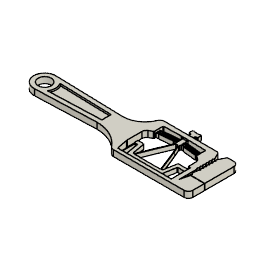
Final_BinaryStiffnessWrench (Autodesk Fusion 360 design; units mm, degrees)
Autodesk Fusion 360 part; units mm, degrees
note: some values were not read from the file. Set by a fixed rule: which sketch regions a step uses.
(part 1 of 3)
sketch "Sketch1" plane through (0, 0, 0) normal (0, 0, 1) x (1, 0, 0)
  arc A0 (89.3732, 10.2649) -> (113.1229, 26.2409) centre (89.45, 35.7917) ccw
  arc A1 (11.704, 12.452) -> (11.9433, -12.5645) centre (11.002, -0.0641) ccw
  arc A2 (112.7407, -25.7315) -> (80.6073, -9.9709) centre (80.1774, -51.4853) ccw
  line L0 (176.5, -1.6298) -> (183.1113, -1.6298)
  line L1 (184, 5.6067) -> (184, 5.6087)
  line L2 (149.0449, 22.5392) -> (149.0454, 22.5392)
  line L3 (184.0001, 9.0708) -> (184.0001, 9.073)
  line L4 (172.4, -5.8471) -> (172.4, -5.8496)
  line L5 (177.088, -7.1298) -> (177.088, -23.1298)
  line L6 (177.588, -23.1298) -> (177.588, -7.1298)
  line L7 (202.169, -22.6429) -> (202.2039, -9.25)
  circle A3 centre (11.002, -0.0641) radius 7.5
  line L8 (11.9433, -12.5645) -> (80.6073, -9.9709)
  line L9 (202.156, -8.9998) -> (202.156, 24.3702)
  line L10 (89.3732, 10.2649) -> (11.704, 12.452)
  line L11 (121.2059, -23.1298) -> (121.2059, -7.1298)
  line L12 (171.2956, -5.8495) -> (171.2956, -5.8471)
  line L13 (184, 2.1426) -> (184, 2.1446)
  line L14 (186.578, -8.932) -> (202.156, -8.9998)
  line L15 (184.001, 12.5353) -> (184.001, 12.5385)
  line L16 (186.1089, -9.5607) -> (182.6828, -23.2512)
  line L17 (202.2039, -9.25) -> (186.5961, -9.1821)
  line L18 (177.588, -28.2111) -> (177.588, -28.4)
  spline S0 degree 3 poles (139.0353, -28.3354) (139.0353, -28.3354) (139.0354, -28.3354) (139.0354, -28.3354) knots 113.159202 113.159202 113.159202 113.159202 113.159512 113.159512 113.159512 113.159512
  line L19 (169.6572, 23.9078) -> (150.1207, 24.3589)
  line L20 (149.6323, 24.8588) -> (149.6323, 29.3702)
  line L21 (149.6323, 29.3702) -> (178.1615, 29.3702)
  line L22 (178.088, -23.6298) -> (182.1978, -23.6298)
  line L23 (169.2352, -6.6298) -> (176.588, -6.6298)
  line L24 (121.7059, -6.6298) -> (122.93, -6.6298)
  line L25 (120.2059, -2.6298) -> (126.2864, -2.6298)
  line L26 (126.0097, -21.7167) -> (123.4224, -7.043)
  line L27 (168.7428, -7.043) -> (166.1554, -21.7167)
  spline S1 degree 5 poles (159.9652, -15.6911) (159.8529, -15.3927) (159.4459, -14.3123) (158.7459, -12.4635) (157.7568, -9.8732) (156.4844, -6.5848) (155.0461, -2.9325) (153.6231, 0.6091) (152.4351, 3.5002) (151.5369, 5.6459) (150.9212, 7.0983) (150.5836, 7.8891) (150.5222, 8.0328) knots 0.061951 0.061951 0.061951 0.061951 0.061951 0.061951 0.1 0.2 0.3 0.4 0.5 0.6 0.7 0.722257 0.722257 0.722257 0.722257 0.722257 0.722257
  line L28 (132.1188, -18.1298) -> (160.1605, -18.1298)
  line L29 (159.9652, -15.6911) -> (160.6285, -17.4538)
  line L30 (126.5021, -22.1298) -> (165.663, -22.1298)
  line L31 (119.7059, -3.1298) -> (119.7059, -6.1298)
  line L32 (120.2059, -23.6298) -> (118.121, -23.6298)
  line L33 (121.7059, -23.6298) -> (176.588, -23.6298)
  line L34 (120.7059, -7.1298) -> (120.7059, -23.1298)
  line L35 (170.1456, 15.3966) -> (193.3883, 15.3966) construction
  line L36 (146.1323, 17.0362) -> (146.1323, 33.8702) construction
  line L37 (170.1456, 15.8966) -> (192.9161, 15.8966) construction
  line L38 (170.1456, 17.3966) -> (193.3497, 17.3966) construction
  line L39 (170.1456, 17.2165) -> (170.1456, 16.1187)
  line L40 (170.1456, 17.8966) -> (193.2684, 17.8966) construction
  line L41 (170.1456, 18.1187) -> (170.1456, 19.2165)
  line L42 (186.7149, 19.4345) -> (191.4009, 19.4345) construction
  line L43 (170.1456, 20.1187) -> (170.1456, 23.408)
  line L44 (148.6323, 17.4356) -> (148.6323, 15.55)
  line L45 (148.6323, 19.4356) -> (148.6323, 18.3378)
  line L46 (148.6323, 33.3702) -> (148.6323, 22.3378)
  line L47 (148.6323, 21.4356) -> (148.6323, 20.3378)
  line L48 (170.1456, 15.2165) -> (170.1456, 13.9739)
  line L49 (170.6456, 13.1079) -> (173.5, 11.4599)
  spline S2 degree 5 poles (130.7595, -17.6378) (131.012, -16.9513) (131.5314, -15.5453) (132.3224, -13.424) (133.3923, -10.5941) (134.7528, -7.0662) (136.1486, -3.5243) (137.5684, -0.0041) (139.0131, 3.4934) (140.482, 6.9691) (141.8006, 10.0246) (142.8329, 12.3782) (143.5692, 14.0387) (144.0034, 15.0117) (144.1323, 15.3) knots 0.004792 0.004792 0.004792 0.004792 0.004792 0.004792 0.1 0.2 0.3 0.4 0.5 0.6 0.7 0.8 0.9 0.94214 0.94214 0.94214 0.94214 0.94214 0.94214
  spline S3 degree 5 poles (144.9323, 15.3) (144.7729, 14.9268) (144.3238, 13.8732) (143.5856, 12.1354) (142.5604, 9.7063) (141.2507, 6.5745) (139.8173, 3.108) (138.3903, -0.385) (136.9701, -3.9054) (135.5564, -7.4521) (134.2095, -10.8681) (133.1481, -13.5859) (132.3693, -15.5934) (131.871, -16.8829) (131.6523, -17.4499) knots 0.045074 0.045074 0.045074 0.045074 0.045074 0.045074 0.1 0.2 0.3 0.4 0.5 0.6 0.7 0.8 0.9 0.978339 0.978339 0.978339 0.978339 0.978339 0.978339
  spline S4 degree 3 poles (150.5222, 8.0328) (150.3157, 8.4943) (150.1094, 8.9559) (149.9035, 9.4176) (149.4682, 10.3932) (149.0343, 11.3694) (148.603, 12.3469) (148.2003, 13.2596) (147.7999, 14.1733) (147.4174, 15.0945) (147.3889, 15.163) (147.3606, 15.2315) (147.3323, 15.3) knots -96.269727 -96.269727 -96.269727 -96.269727 -93.23622 -93.23622 -93.23622 -86.826165 -86.826165 -86.826165 -80.841267 -80.841267 -80.841267 -80.396364 -80.396364 -80.396364 -80.396364
  line L50 (143.6323, 33.3702) -> (143.6323, 22.3378)
  line L51 (143.6323, 21.4356) -> (143.6323, 20.3378)
  line L52 (143.6323, 19.4356) -> (143.6323, 18.3378)
  line L53 (143.6323, 17.4356) -> (143.6323, 15.55)
  line L54 (122.1189, 17.2165) -> (122.1189, 16.1187)
  line L55 (122.1189, 18.1187) -> (122.1189, 19.2165)
  line L56 (122.1189, 20.1187) -> (122.1189, 23.408)
  line L57 (122.1189, 15.2165) -> (122.1189, 13.9739)
  line L58 (142.6323, 29.3702) -> (117.7597, 29.3702)
  line L59 (143.8823, 15.3) -> (144.1323, 15.3)
  line L60 (144.9323, 15.3) -> (147.3323, 15.3)
  line L61 (148.1323, 15.3) -> (148.3823, 15.3)
  line L62 (130.7595, -17.6378) -> (129.7718, -17.6378)
  line L63 (129.2794, -17.2246) -> (126.7788, -3.043)
  line L64 (162.9139, -17.0652) -> (165.3864, -3.043)
  line L65 (165.8788, -2.6298) -> (184.9592, -2.6298)
  line L66 (185.4592, 0) -> (185.4592, -2.1298)
  line L67 (117.6907, 10.8399) -> (121.6189, 13.1079)
  line L68 (151.6323, 22.1424) -> (167.1456, 20.5119)
  line L69 (151.6323, 21.0424) -> (167.1456, 19.4119)
  line L70 (151.6323, 20.1424) -> (167.1456, 18.5119)
  line L71 (151.6323, 19.0424) -> (167.1456, 17.4119)
  line L72 (151.6323, 18.1424) -> (167.1456, 16.5119)
  line L73 (151.6323, 17.0424) -> (167.1456, 15.4119)
  line L74 (169.9247, 19.9198) -> (167.3247, 20.1931)
  line L75 (151.4114, 21.8656) -> (148.8114, 22.1389)
  line L76 (169.9665, 19.4154) -> (167.3665, 19.6887)
  line L77 (151.4532, 21.3612) -> (148.8532, 21.6345)
  line L78 (151.6323, 22.1424) -> (151.6323, 22.0645)
  line L79 (151.6323, 21.1623) -> (151.6323, 21.0424)
  line L80 (151.6323, 20.1424) -> (151.6323, 20.0645)
  line L81 (151.6323, 19.1623) -> (151.6323, 19.0424)
  line L82 (169.9665, 17.4154) -> (167.3665, 17.6887)
  line L83 (151.4532, 19.3612) -> (148.8532, 19.6345)
  line L84 (169.9247, 17.9198) -> (167.3247, 18.1931)
  line L85 (151.4114, 19.8656) -> (148.8114, 20.1389)
  line L86 (151.6323, 18.1424) -> (151.6323, 18.0645)
  line L87 (151.6323, 17.1623) -> (151.6323, 17.0424)
  line L88 (169.9665, 15.4154) -> (167.3665, 15.6887)
  line L89 (151.4532, 17.3612) -> (148.8532, 17.6345)
  line L90 (169.9247, 15.9198) -> (167.3247, 16.1931)
  line L91 (151.4114, 17.8656) -> (148.8114, 18.1389)
  line L92 (167.1456, 20.5119) -> (167.1456, 20.392)
  line L93 (167.1456, 19.4898) -> (167.1456, 19.4119)
  line L94 (167.1456, 18.5119) -> (167.1456, 18.392)
  line L95 (167.1456, 17.4898) -> (167.1456, 17.4119)
  line L96 (167.1456, 16.5119) -> (167.1456, 16.392)
  line L97 (167.1456, 15.4898) -> (167.1456, 15.4119)
  line L98 (140.6323, 17.1623) -> (140.6323, 17.2225)
  line L99 (140.6323, 21.2524) -> (140.6323, 21.2225)
  line L100 (140.7218, 19.3518) -> (143.4114, 19.6345)
  line L101 (140.6323, 19.8424) -> (143.4532, 20.1389)
  line L102 (140.6323, 17.9203) -> (140.6323, 17.8424)
  line L103 (140.4532, 17.0236) -> (125.3398, 15.4351)
  line L104 (122.3398, 15.9198) -> (125.1189, 16.2119)
  line L105 (140.6323, 19.2524) -> (140.6323, 19.2225)
  line L106 (140.4532, 19.0236) -> (125.3398, 17.4351)
  line L107 (140.4532, 21.0236) -> (125.3398, 19.4351)
  line L108 (140.6323, 21.8424) -> (143.4532, 22.1389)
  line L109 (125.1189, 17.7119) -> (125.1189, 17.634)
  line L110 (122.3398, 19.9198) -> (125.0294, 20.2025)
  line L111 (140.7218, 21.3518) -> (143.4114, 21.6345)
  line L112 (140.8114, 17.3612) -> (143.4114, 17.6345)
  line L113 (125.1189, 15.7119) -> (125.1189, 15.634)
  line L114 (122.298, 17.4154) -> (125.1189, 17.7119)
  line L115 (140.4114, 22.1192) -> (125.298, 20.5307)
  line L116 (140.4114, 20.1192) -> (125.298, 18.5307)
  line L117 (140.4114, 18.1192) -> (125.298, 16.5307)
  line L118 (122.3398, 17.9198) -> (125.1189, 18.2119)
  line L119 (125.1189, 16.3318) -> (125.1189, 16.2119)
  line L120 (140.6323, 17.8424) -> (143.4532, 18.1389)
  line L121 (122.298, 19.4154) -> (125.1189, 19.7119)
  line L122 (125.1189, 18.3318) -> (125.1189, 18.2119)
  line L123 (125.1189, 19.7119) -> (125.1189, 19.634)
  line L124 (140.6323, 19.9203) -> (140.6323, 19.8424)
  line L125 (122.298, 15.4154) -> (125.1189, 15.7119)
  line L126 (125.1189, 20.3318) -> (125.1189, 20.3019)
  line L127 (140.6323, 21.9203) -> (140.6323, 21.8424)
  line L128 (115.1907, 6.5098) -> (115.1907, -10.1247)
  line L129 (117.6301, -23.2247) -> (115.2816, -11.0735)
  line L130 (178.088, -6.6298) -> (185.5859, -6.6298)
  line L131 (186.0859, -7.132) -> (186.0802, -8.4298)
  line L132 (116.6624, -27.6298) -> (197.169, -27.6298)
  line L133 (142.6323, 29.3702) -> (142.6323, 24.8588)
  line L134 (142.1438, 24.3589) -> (122.6074, 23.9078)
  line L135 (162.4215, -17.4784) -> (161.7176, -17.4784)
  spline S5 degree 5 poles (148.1323, 15.3) (148.4158, 14.6516) (148.9812, 13.354) (149.8244, 11.4057) (150.9388, 8.8038) (152.3141, 5.5444) (153.6703, 2.2771) (155.0058, -0.9987) (156.3196, -4.2834) (157.6127, -7.5765) (158.8598, -10.8079) (159.8388, -13.3845) (160.5594, -15.3025) (161.0282, -16.559) (161.2489, -17.1526) knots 0 0 0 0 0 0 0.1 0.2 0.3 0.4 0.5 0.6 0.7 0.8 0.9 0.989467 0.989467 0.989467 0.989467 0.989467 0.989467
  line L136 (190.889, 29.3702) -> (197.156, 29.3702)
  line L137 (183.6113, 17.3326) -> (182.6113, 15.6006)
  line L138 (182.6113, 15.6006) -> (183.6113, 13.8685)
  line L139 (183.6113, 13.8685) -> (182.6113, 12.1365)
  line L140 (182.6113, 12.1365) -> (183.6113, 10.4044)
  line L141 (183.6113, 10.4044) -> (182.6113, 8.6724)
  line L142 (182.6113, 8.6724) -> (183.6113, 6.9403)
  line L143 (183.6113, 6.9403) -> (182.6113, 5.2083)
  line L144 (182.6113, 5.2083) -> (183.6113, 3.4762)
  line L145 (183.6113, 3.4762) -> (182.6113, 1.7442)
  line L146 (182.6113, 1.7442) -> (183.6113, 0.0121)
  line L147 (183.6113, 0.0121) -> (183.6113, -1.1298)
  line L148 (183.6113, 17.3326) -> (182.6113, 19.0647)
  line L149 (183.6113, 17.3326) -> (185.8426, 17.3326) construction
  line L150 (182.6113, 19.0647) -> (183.6113, 20.7967)
  line L151 (182.6113, 19.0647) -> (184.8426, 19.0647) construction
  line L152 (183.6113, 20.7967) -> (179.9574, 28.2505)
  line L153 (176, 7.1298) -> (176, -1.1298)
  line L154 (184.5253, -0.9908) -> (184.5253, 23.394) construction
  line L155 (186.4393, 19.0647) -> (185.4393, 20.7967)
  line L156 (185.4393, 20.7967) -> (189.0932, 28.2505)
  line L157 (185.4393, 17.3326) -> (186.4393, 19.0647)
  line L158 (185.4393, 17.3326) -> (186.4393, 15.6006)
  line L159 (186.4393, 15.6006) -> (185.4393, 13.8685)
  line L160 (185.4393, 13.8685) -> (186.4393, 12.1365)
  line L161 (186.4393, 12.1365) -> (185.4393, 10.4044)
  line L162 (185.4393, 10.4044) -> (186.4393, 8.6724)
  line L163 (186.4393, 8.6724) -> (185.4393, 6.9403)
  line L164 (185.4393, 6.9403) -> (186.4393, 5.2083)
  line L165 (186.4393, 5.2083) -> (185.4393, 3.4762)
  line L166 (185.4393, 3.4762) -> (186.4393, 1.7442)
  line L167 (186.4393, 1.7442) -> (185.4592, 0.0467)
  line L168 (185.4592, 0) -> (185.4592, 0.0467)
  arc A4 (122.6074, 23.9078) -> (122.1189, 23.408) centre (122.6189, 23.408) ccw
  arc A5 (170.1456, 23.408) -> (169.6572, 23.9078) centre (169.6456, 23.408) ccw
  arc A6 (170.1456, 13.9739) -> (170.6456, 13.1079) centre (171.1456, 13.9739) ccw
  arc A7 (176, 7.1298) -> (173.5, 11.4599) centre (171, 7.1298) ccw
  arc A8 (121.6189, 13.1079) -> (122.1189, 13.9739) centre (121.1189, 13.9739) ccw
  arc A9 (117.6907, 10.8399) -> (115.1907, 6.5098) centre (120.1907, 6.5098) ccw
  arc A10 (117.6301, -23.2247) -> (118.121, -23.6298) centre (118.121, -23.1298) ccw
  arc A11 (120.2059, -23.6298) -> (120.7059, -23.1298) centre (120.2059, -23.1298) ccw
  arc A12 (121.2059, -23.1298) -> (121.7059, -23.6298) centre (121.7059, -23.1298) ccw
  arc A13 (176.588, -23.6298) -> (177.088, -23.1298) centre (176.588, -23.1298) ccw
  arc A14 (177.588, -23.1298) -> (178.088, -23.6298) centre (178.088, -23.1298) ccw
  arc A15 (182.1978, -23.6298) -> (182.6828, -23.2512) centre (182.1978, -23.1298) ccw
  arc A16 (178.088, -6.6298) -> (177.588, -7.1298) centre (178.088, -7.1298) ccw
  arc A17 (177.088, -7.1298) -> (176.588, -6.6298) centre (176.588, -7.1298) ccw
  arc A18 (169.2352, -6.6298) -> (168.7428, -7.043) centre (169.2352, -7.1298) ccw
  arc A19 (165.663, -22.1298) -> (166.1554, -21.7167) centre (165.663, -21.6298) ccw
  arc A20 (165.8788, -2.6298) -> (165.3864, -3.043) centre (165.8788, -3.1298) ccw
  arc A21 (162.4215, -17.4784) -> (162.9139, -17.0652) centre (162.4215, -16.9784) ccw
  arc A22 (161.2489, -17.1526) -> (161.7176, -17.4784) centre (161.7176, -16.9784) ccw
  arc A23 (160.1605, -18.1298) -> (160.6285, -17.4538) centre (160.1605, -17.6298) ccw
  arc A24 (131.6523, -17.4499) -> (132.1188, -18.1298) centre (132.1188, -17.6298) ccw
  arc A25 (129.2794, -17.2246) -> (129.7718, -17.6378) centre (129.7718, -17.1378) ccw
  arc A26 (126.7788, -3.043) -> (126.2864, -2.6298) centre (126.2864, -3.1298) ccw
  arc A27 (120.2059, -2.6298) -> (119.7059, -3.1298) centre (120.2059, -3.1298) ccw
  arc A28 (119.7059, -6.1298) -> (120.2059, -6.6298) centre (120.2059, -6.1298) ccw
  arc A29 (120.7059, -7.1298) -> (120.2059, -6.6298) centre (120.2059, -7.1298) ccw
  arc A30 (121.7059, -6.6298) -> (121.2059, -7.1298) centre (121.7059, -7.1298) ccw
  arc A31 (123.4224, -7.043) -> (122.93, -6.6298) centre (122.93, -7.1298) ccw
  arc A32 (126.0097, -21.7167) -> (126.5021, -22.1298) centre (126.5021, -21.6298) ccw
  arc A33 (143.6323, 15.55) -> (143.8823, 15.3) centre (143.8823, 15.55) ccw
  arc A34 (148.3823, 15.3) -> (148.6323, 15.55) centre (148.3823, 15.55) ccw
  arc A35 (125.298, 20.5307) -> (125.1189, 20.3318) centre (125.3189, 20.3318) ccw
  arc A36 (140.6323, 21.9203) -> (140.4114, 22.1192) centre (140.4323, 21.9203) ccw
  arc A37 (140.4532, 21.0236) -> (140.6323, 21.2225) centre (140.4323, 21.2225) ccw
  arc A38 (125.1189, 19.634) -> (125.3398, 19.4351) centre (125.3189, 19.634) ccw
  arc A39 (125.298, 18.5307) -> (125.1189, 18.3318) centre (125.3189, 18.3318) ccw
  arc A40 (125.1189, 17.634) -> (125.3398, 17.4351) centre (125.3189, 17.634) ccw
  arc A41 (140.4532, 19.0236) -> (140.6323, 19.2225) centre (140.4323, 19.2225) ccw
  arc A42 (140.6323, 19.9203) -> (140.4114, 20.1192) centre (140.4323, 19.9203) ccw
  arc A43 (125.298, 16.5307) -> (125.1189, 16.3318) centre (125.3189, 16.3318) ccw
  arc A44 (125.1189, 15.634) -> (125.3398, 15.4351) centre (125.3189, 15.634) ccw
  arc A45 (140.4532, 17.0236) -> (140.6323, 17.2225) centre (140.4323, 17.2225) ccw
  arc A46 (140.6323, 17.9203) -> (140.4114, 18.1192) centre (140.4323, 17.9203) ccw
  arc A47 (122.298, 15.4154) -> (122.1189, 15.2165) centre (122.3189, 15.2165) ccw
  arc A48 (122.1189, 16.1187) -> (122.3398, 15.9198) centre (122.3189, 16.1187) ccw
  arc A49 (122.298, 17.4154) -> (122.1189, 17.2165) centre (122.3189, 17.2165) ccw
  arc A50 (122.1189, 18.1187) -> (122.3398, 17.9198) centre (122.3189, 18.1187) ccw
  arc A51 (122.298, 19.4154) -> (122.1189, 19.2165) centre (122.3189, 19.2165) ccw
  arc A52 (122.1189, 20.1187) -> (122.3398, 19.9198) centre (122.3189, 20.1187) ccw
  arc A53 (143.4532, 22.1389) -> (143.6323, 22.3378) centre (143.4323, 22.3378) ccw
  arc A54 (143.6323, 21.4356) -> (143.4114, 21.6345) centre (143.4323, 21.4356) ccw
  arc A55 (143.4532, 20.1389) -> (143.6323, 20.3378) centre (143.4323, 20.3378) ccw
  arc A56 (143.6323, 19.4356) -> (143.4114, 19.6345) centre (143.4323, 19.4356) ccw
  arc A57 (143.4532, 18.1389) -> (143.6323, 18.3378) centre (143.4323, 18.3378) ccw
  arc A58 (143.6323, 17.4356) -> (143.4114, 17.6345) centre (143.4323, 17.4356) ccw
  arc A59 (140.8114, 17.3612) -> (140.6323, 17.1623) centre (140.8323, 17.1623) ccw
  arc A60 (140.7218, 19.3518) -> (140.6323, 19.2524) centre (140.7323, 19.2524) ccw
  arc A61 (140.7218, 21.3518) -> (140.6323, 21.2524) centre (140.7323, 21.2524) ccw
  arc A62 (125.0294, 20.2025) -> (125.1189, 20.3019) centre (125.0189, 20.3019) ccw
  arc A63 (148.6323, 22.3378) -> (148.8114, 22.1389) centre (148.8323, 22.3378) ccw
  arc A64 (148.8532, 21.6345) -> (148.6323, 21.4356) centre (148.8323, 21.4356) ccw
  arc A65 (148.6323, 20.3378) -> (148.8114, 20.1389) centre (148.8323, 20.3378) ccw
  arc A66 (148.8532, 19.6345) -> (148.6323, 19.4356) centre (148.8323, 19.4356) ccw
  arc A67 (148.6323, 18.3378) -> (148.8114, 18.1389) centre (148.8323, 18.3378) ccw
  arc A68 (148.8532, 17.6345) -> (148.6323, 17.4356) centre (148.8323, 17.4356) ccw
  arc A69 (151.6323, 17.1623) -> (151.4532, 17.3612) centre (151.4323, 17.1623) ccw
  arc A70 (151.4114, 17.8656) -> (151.6323, 18.0645) centre (151.4323, 18.0645) ccw
  arc A71 (151.6323, 19.1623) -> (151.4532, 19.3612) centre (151.4323, 19.1623) ccw
  arc A72 (151.4114, 19.8656) -> (151.6323, 20.0645) centre (151.4323, 20.0645) ccw
  arc A73 (151.6323, 21.1623) -> (151.4532, 21.3612) centre (151.4323, 21.1623) ccw
  arc A74 (151.4114, 21.8656) -> (151.6323, 22.0645) centre (151.4323, 22.0645) ccw
  arc A75 (167.1456, 20.392) -> (167.3247, 20.1931) centre (167.3456, 20.392) ccw
  arc A76 (167.3665, 19.6887) -> (167.1456, 19.4898) centre (167.3456, 19.4898) ccw
  arc A77 (167.1456, 18.392) -> (167.3247, 18.1931) centre (167.3456, 18.392) ccw
  arc A78 (167.3665, 17.6887) -> (167.1456, 17.4898) centre (167.3456, 17.4898) ccw
  arc A79 (167.1456, 16.392) -> (167.3247, 16.1931) centre (167.3456, 16.392) ccw
  arc A80 (167.3665, 15.6887) -> (167.1456, 15.4898) centre (167.3456, 15.4898) ccw
  arc A81 (170.1456, 19.2165) -> (169.9665, 19.4154) centre (169.9456, 19.2165) ccw
  arc A82 (169.9247, 19.9198) -> (170.1456, 20.1187) centre (169.9456, 20.1187) ccw
  arc A83 (169.9247, 17.9198) -> (170.1456, 18.1187) centre (169.9456, 18.1187) ccw
  arc A84 (170.1456, 17.2165) -> (169.9665, 17.4154) centre (169.9456, 17.2165) ccw
  arc A85 (169.9247, 15.9198) -> (170.1456, 16.1187) centre (169.9456, 16.1187) ccw
  arc A86 (170.1456, 15.2165) -> (169.9665, 15.4154) centre (169.9456, 15.2165) ccw
  arc A87 (117.7597, 29.3702) -> (113.1229, 26.2409) centre (117.7597, 24.3702) ccw
  arc A88 (112.7407, -25.7315) -> (116.6624, -27.6298) centre (116.6624, -22.6298) ccw
  arc A89 (202.156, 24.3702) -> (197.156, 29.3702) centre (197.156, 24.3702) ccw
  arc A90 (197.169, -27.6298) -> (202.169, -22.6429) centre (197.169, -22.6298) ccw
  arc A91 (184.9592, -2.6298) -> (185.4592, -2.1298) centre (184.9592, -2.1298) ccw
  arc A92 (186.0859, -7.132) -> (185.5859, -6.6298) centre (185.5859, -7.1298) ccw
  arc A93 (186.0802, -8.4298) -> (186.578, -8.932) centre (186.5802, -8.432) ccw
  arc A94 (186.5961, -9.1821) -> (186.1089, -9.5607) centre (186.5939, -9.6821) ccw
  arc A95 (179.9574, 28.2505) -> (178.1615, 29.3702) centre (178.1615, 27.3702) ccw
  arc A96 (190.889, 29.3702) -> (189.0932, 28.2505) centre (190.889, 27.3702) ccw
  line L169 (149.1323, 33.8702) -> (150.6323, 33.8702)
  line L170 (143.1323, 33.8702) -> (141.6323, 33.8702)
  line L171 (141.1323, 34.3702) -> (141.1323, 38.0378)
  line L172 (151.1323, 34.3702) -> (151.1323, 38.0378)
  arc A97 (141.7774, 38.5162) -> (150.4871, 38.5162) centre (146.1323, 52.8702) ccw
  arc A98 (143.6323, 33.3702) -> (143.1323, 33.8702) centre (143.1323, 33.3702) ccw
  arc A99 (141.1323, 34.3702) -> (141.6323, 33.8702) centre (141.6323, 34.3702) ccw
  arc A100 (149.1323, 33.8702) -> (148.6323, 33.3702) centre (149.1323, 33.3702) ccw
  arc A101 (150.6323, 33.8702) -> (151.1323, 34.3702) centre (150.6323, 34.3702) ccw
  arc A102 (151.1323, 38.0378) -> (150.4871, 38.5162) centre (150.6323, 38.0378) ccw
  arc A103 (141.7774, 38.5162) -> (141.1323, 38.0378) centre (141.6323, 38.0378) ccw
  line L173 (142.6323, 24.8588) -> (142.6323, 24.3589)
  line L174 (149.6323, 24.8588) -> (149.6323, 24.3702)
  line L175 (150.1207, 24.3589) -> (149.6323, 24.3702)
  line L176 (142.1438, 24.3589) -> (142.6323, 24.3589)
  line L177 (176.5, -1.6298) -> (176, -1.6298)
  line L178 (183.1113, -1.6298) -> (183.6113, -1.6298)
  line L179 (176, -1.1298) -> (176, -1.6298)
  line L180 (183.6113, -1.1298) -> (183.6113, -1.6298)
  arc A104 (115.1907, -10.1247) -> (115.2816, -11.0735) centre (120.1907, -10.1247) ccw
  point P0 (114.156, 29.3702)
  point P1 (186.204, -9.1804)
  point P2 (114.156, -27.6298)
  point P3 (177.588, -6.6298)
  point P4 (131.3903, -18.1298)
  point P5 (121.2059, -6.6298)
  point P6 (166.0826, -22.1298)
  point P7 (115.1907, 9.3966)
  point P8 (177.088, -23.6298)
  point P9 (177.588, -23.6298)
  point P10 (182.588, -23.6298)
  point P11 (121.2059, -23.6298)
  point P12 (177.088, -6.6298)
  point P13 (119.7059, -2.6298)
  point P14 (126.7059, -2.6298)
  point P15 (126.0826, -22.1298)
  point P16 (119.7059, -6.6298)
  point P17 (120.7059, -6.6298)
  point P18 (117.7084, -23.6298)
  point P19 (120.7084, -23.6298)
  point P20 (120.7059, -23.6298)
  point P21 (148.6323, 33.8702)
  point P22 (148.6323, 15.3)
  point P23 (170.1456, 19.3966)
  point P24 (170.1456, 23.8966)
  point P25 (170.1456, 19.8966)
  point P26 (170.1456, 13.3966)
  point P27 (143.6323, 33.8702)
  point P28 (143.6323, 15.3)
  point P29 (122.1189, 13.3966)
  point P30 (129.3522, -17.6378)
  point P31 (165.4592, -2.6298)
  point P32 (185.4592, -2.6298)
  point P33 (167.1456, 20.2119)
  point P34 (151.6323, 21.8424)
  point P35 (167.1456, 19.7119)
  point P36 (151.6323, 19.8424)
  point P37 (151.6323, 19.3424)
  point P38 (151.6323, 17.8424)
  point P39 (151.6323, 17.3424)
  point P40 (115.1907, -10.6034)
  point P41 (186.088, -6.6298)
  point P42 (186.078, -8.9298)
  point P43 (202.156, -27.6298)
  point P44 (142.6323, 24.3702)
  point P45 (155, -1)
  point P46 (151.1323, 33.8702)
  point P47 (141.1323, 33.8702)
  dimension "d4" = 5
  dimension "d16" = 40
  dimension "d19" = 4
  dimension "d21" = 1.5
  dimension "d22" = 0.5
  dimension "d24" = 17
  dimension "d25" = 17
  dimension "d27" = 17
  dimension "d28" = 17
  dimension "d29" = 17
  dimension "d30" = 0.5
  dimension "d31" = 0.8
  dimension "d33" = 174
  dimension "d34" = 2.5
  dimension "d35" = 174
  dimension "d36" = 174
  dimension "d37" = 174
  dimension "d38" = 96
  dimension "d39" = 0.5
  dimension "d40" = 1.5
  dimension "d41" = 0.5
  dimension "d42" = 1.5
  dimension "d43" = 174
  dimension "d44" = 0.5
  dimension "d46" = 4
  dimension "d47" = 2
  dimension "d49" = 1
  dimension "d50" = 0.8
  dimension "d51" = 0.5
  dimension "d52" = 0.8
  dimension "d53" = 0.5
  dimension "d54" = 100
  dimension "d55" = 100
  dimension "d57" = 4
  dimension "d58" = 1
  dimension "d60" = 90
  dimension "d61" = 4
  dimension "d62" = 4
  dimension "d63" = 3
  dimension "d64" = 3
  dimension "d65" = 0.3
  dimension "d66" = 0.3
  dimension "d67" = 0.3
  dimension "d68" = 0.3
  dimension "d69" = 0.3
  dimension "d70" = 0.3
  dimension "d71" = 0.3
  dimension "d72" = 8
  dimension "d73" = 120
  dimension "d74" = 20
  dimension "d75" = 3
  dimension "d76" = 5
  dimension "d77" = 0.25
  dimension "d80" = 16
  dimension "d83" = 8.5
  dimension "d84" = 88
  dimension "d85" = 4
  dimension "d86" = 57
  dimension "d87" = 57
  dimension "d88" = 5
  dimension "d89" = 1
  dimension "d90" = 7
  dimension "d96" = 88
  dimension "d97" = 120
  dimension "d98" = 2
  dimension "d99" = 2
  dimension "d100" = 2
  dimension "d101" = 2
  dimension "d102" = 2
  dimension "d103" = 120
  dimension "d104" = 2
  dimension "d105" = 120
  dimension "d106" = 120
  dimension "d107" = 2
  dimension "d108" = 60
  dimension "d109" = 2
  dimension "d110" = 1.848
  dimension "d111" = 20
  dimension "d112" = 4
  dimension "d113" = 2.3
  dimension "d114" = 1
  dimension "d115" = 120
  dimension "d116" = 0.914
  dimension "d118" = 2
  dimension "d119" = 2
  dimension "d120" = 2
  dimension "d121" = 120
  dimension "d122" = 120
  dimension "d123" = 2
  dimension "d124" = 120
  dimension "d125" = 150
  dimension "d127" = 0.5
  dimension "d129" = 0.5
  dimension "d130" = 0.5
  dimension "d131" = 0.5
  dimension "d132" = 0.25
  dimension "d133" = 0.25
  dimension "d134" = 0.2
  dimension "d135" = 0.1
  dimension "d136" = 0.1
  dimension "d137" = 0.1
  dimension "d138" = 0.2
  dimension "d139" = 5
  dimension "d140" = 5
  dimension "d141" = 5
  dimension "d142" = 0.5
  dimension "d143" = 2
  dimension "d145" = 2.5
  dimension "d146" = 2.5
  dimension "d148" = 30
  dimension "d150" = 0.5
  dimension "d164" = 5
  dimension "d165" = 5
  dimension "d166" = 5
  dimension "d167" = 1
  dimension "d168" = 1
  constraint vertical L20
  constraint perpendicular L20 L21
  constraint perpendicular L6 L22
  constraint horizontal L24
  constraint horizontal L28
  constraint perpendicular L25 L31
  constraint perpendicular L11 L33
  constraint perpendicular L32 L34
  constraint coincident L32 P20
  constraint horizontal L35
  constraint horizontal L59
  constraint perpendicular L36 L60
  constraint perpendicular L44 L61
  constraint horizontal L37
  constraint horizontal L38
  constraint perpendicular L38 L39
  constraint horizontal L40
  constraint perpendicular L40 L41
  constraint horizontal L42
  constraint vertical L43
  constraint collinear L44 L45
  constraint collinear L45 L47
  constraint collinear L46 L47
  constraint collinear L41 L43
  constraint collinear L39 L41
  constraint perpendicular L35 L48
  constraint collinear L39 L48
  constraint symmetric L36 P21 P27
  constraint symmetric L36 P22 P28
  constraint symmetric L36 P26 P29
  constraint perpendicular L50 L58
  constraint collinear L59 L60
  constraint collinear L60 L61
  constraint coincident S2.start L62.start
  constraint horizontal L62
  constraint parallel L26 L63
  constraint parallel L27 L64
  constraint horizontal L65
  constraint perpendicular L65 L66
  constraint vertical L78
  constraint vertical L92
  constraint parallel L69 L76
  constraint parallel L70 L85
  constraint parallel L71 L82
  constraint parallel L72 L91
  constraint parallel L73 L88
  constraint collinear L79 L80
  constraint collinear L81 L86
  constraint collinear L95 L96
  constraint collinear L93 L94
  constraint collinear L74 L75
  constraint collinear L76 L77
  constraint collinear L78 L79
  constraint collinear L80 L81
  constraint collinear L82 L83
  constraint collinear L84 L85
  constraint collinear L86 L87
  constraint collinear L88 L89
  constraint collinear L90 L91
  constraint collinear L92 L93
  constraint collinear L94 L95
  constraint collinear L96 L97
  constraint symmetric L36 P34 L108.start
  constraint symmetric L36 P35 L121.end
  constraint symmetric L36 P36 L101.start
  constraint symmetric L36 P38 L102.end
  constraint vertical L128
  constraint perpendicular L6 L130
  constraint perpendicular L14 L131
  constraint horizontal L132
  constraint perpendicular L58 L133
  constraint horizontal L135
  constraint vertical L9
  constraint parallel L21 L136
  constraint parallel L142 L144
  constraint parallel L143 L145
  constraint parallel L144 L146
  constraint perpendicular L0 L147
  constraint horizontal L149
  constraint horizontal L151
  constraint perpendicular L0 L153
  constraint perpendicular L149 L154
  constraint symmetric L137.start L154 L157.start
  constraint symmetric L145.end L154 L166.end
  constraint symmetric L144.end L154 L165.end
  constraint symmetric L143.end L154 L164.end
  constraint symmetric L137.end L154 L158.end
  constraint symmetric L138.end L154 L159.end
  constraint symmetric L139.end L154 L160.end
  constraint symmetric L141.end L154 L162.end
  constraint symmetric L142.end L154 L163.end
  constraint symmetric L140.end L154 L161.end
  constraint symmetric L148.end L154 L155.start
  constraint symmetric L150.end L154 L155.end
  constraint parallel L66 L168
  constraint tangent L56 A4
  constraint tangent L134 A4
  constraint coincident P44 L133
  constraint coincident P44 L134
  constraint coincident L174.end L19
  constraint coincident L174.end L20
  constraint coincident L43 P24
  constraint coincident L19 P24
  constraint tangent L43 A5
  constraint tangent L19 A5
  constraint coincident P26 L48
  constraint coincident P26 L49
  constraint tangent L48 A6
  constraint tangent L49 A6
  constraint tangent L49 A7
  constraint tangent L153 A7
  constraint coincident P29 L57
  constraint coincident P29 L67
  constraint tangent L57 A8
  constraint tangent L67 A8
  constraint coincident P7 L67
  constraint coincident P7 L128
  constraint tangent L67 A9
  constraint tangent L128 A9
  constraint coincident L32 P18
  constraint coincident P18 L129
  constraint tangent L32 A10
  constraint tangent L129 A10
  constraint coincident L34 P20
  constraint tangent L34 A11
  constraint tangent L32 A11
  constraint coincident L11 P11
  constraint coincident P11 L33
  constraint tangent L11 A12
  constraint tangent L33 A12
  constraint coincident L5 P8
  constraint tangent L5 A13
  constraint tangent L33 A13
  constraint coincident L6 P9
  constraint coincident P9 L22
  constraint tangent L6 A14
  constraint tangent L22 A14
  constraint coincident L16 P10
  constraint coincident P10 L22
  constraint tangent L16 A15
  constraint tangent L22 A15
  constraint coincident P3 L6
  constraint coincident P3 L130
  constraint tangent L6 A16
  constraint tangent L130 A16
  constraint coincident L5 P12
  constraint coincident P12 L23
  constraint tangent L5 A17
  constraint tangent L23 A17
  constraint tangent L23 A18
  constraint tangent L27 A18
  constraint coincident P6 L27
  constraint coincident P6 L30
  constraint tangent L27 A19
  constraint tangent L30 A19
  constraint coincident P31 L64
  constraint coincident P31 L65
  constraint tangent L64 A20
  constraint tangent L65 A20
  constraint tangent L64 A21
  constraint tangent L135 A21
  constraint tangent L135 A22
  constraint tangent S5 A22
  constraint tangent L28 A23
  constraint tangent L29 A23
  constraint tangent L28 A24
  constraint tangent S3 A24
  constraint coincident P30 L62
  constraint coincident P30 L63
  constraint tangent L62 A25
  constraint tangent L63 A25
  constraint coincident P14 L25
  constraint coincident P14 L63
  constraint tangent L25 A26
  constraint tangent L63 A26
  constraint coincident P13 L25
  constraint coincident P13 L31
  constraint tangent L25 A27
  constraint tangent L31 A27
  constraint coincident P16 L31
  constraint tangent L31 A28
  constraint equal A27 A28
  constraint coincident P17 L34
  constraint tangent L34 A29
  constraint equal A27 A29
  constraint coincident A28.end A29.end
  constraint coincident P5 L11
  constraint coincident P5 L24
  constraint tangent L11 A30
  constraint tangent L24 A30
  constraint equal A27 A30
  constraint tangent L26 A31
  constraint tangent L24 A31
  constraint equal A27 A31
  constraint coincident P15 L26
  constraint coincident P15 L30
  constraint tangent L26 A32
  constraint tangent L30 A32
  constraint coincident P28 L53
  constraint tangent L53 A33
  constraint tangent L59 A33
  constraint coincident P22 L44
  constraint coincident P22 L61
  constraint tangent L44 A34
  constraint tangent L61 A34
  constraint tangent L115 A35
  constraint tangent L126 A35
  constraint tangent L115 A36
  constraint tangent L127 A36
  constraint equal A35 A36
  constraint tangent L99 A37
  constraint tangent L107 A37
  constraint equal A35 A37
  constraint tangent L107 A38
  constraint tangent L123 A38
  constraint equal A35 A38
  constraint tangent L116 A39
  constraint tangent L122 A39
  constraint equal A35 A39
  constraint tangent L106 A40
  constraint tangent L109 A40
  constraint equal A35 A40
  constraint tangent L105 A41
  constraint tangent L106 A41
  constraint equal A35 A41
  constraint tangent L116 A42
  constraint tangent L124 A42
  constraint equal A35 A42
  constraint tangent L117 A43
  constraint tangent L119 A43
  constraint equal A35 A43
  constraint tangent L103 A44
  constraint tangent L113 A44
  constraint equal A35 A44
  constraint tangent L98 A45
  constraint tangent L103 A45
  constraint equal A35 A45
  constraint tangent L102 A46
  constraint tangent L117 A46
  constraint equal A35 A46
  constraint tangent L57 A47
  constraint tangent L125 A47
  constraint equal A35 A47
  constraint tangent L104 A48
  constraint tangent L54 A48
  constraint equal A35 A48
  constraint tangent L114 A49
  constraint tangent L54 A49
  constraint equal A35 A49
  constraint tangent L118 A50
  constraint tangent L55 A50
  constraint equal A35 A50
  constraint tangent L121 A51
  constraint tangent L55 A51
  constraint equal A35 A51
  constraint tangent L110 A52
  constraint tangent L56 A52
  constraint equal A35 A52
  constraint tangent L108 A53
  constraint tangent L50 A53
  constraint equal A35 A53
  constraint tangent L111 A54
  constraint tangent L51 A54
  constraint equal A35 A54
  constraint tangent L101 A55
  constraint tangent L51 A55
  constraint equal A35 A55
  constraint tangent L100 A56
  constraint tangent L52 A56
  constraint equal A35 A56
  constraint tangent L120 A57
  constraint tangent L52 A57
  constraint equal A35 A57
  constraint tangent L112 A58
  constraint tangent L53 A58
  constraint equal A35 A58
  constraint tangent L98 A59
  constraint tangent L112 A59
  constraint equal A35 A59
  constraint tangent L100 A60
  constraint tangent L105 A60
  constraint tangent L99 A61
  constraint tangent L111 A61
  constraint tangent L110 A62
  constraint tangent L126 A62
  constraint tangent L46 A63
  constraint tangent L75 A63
  constraint tangent L47 A64
  constraint tangent L77 A64
  constraint equal A63 A64
  constraint tangent L47 A65
  constraint tangent L85 A65
  constraint equal A63 A65
  constraint tangent L45 A66
  constraint tangent L83 A66
  constraint equal A63 A66
  constraint tangent L45 A67
  constraint tangent L91 A67
  constraint equal A63 A67
  constraint tangent L44 A68
  constraint tangent L89 A68
  constraint equal A63 A68
  constraint coincident P39 L87
  constraint coincident P39 L89
  constraint tangent L87 A69
  constraint tangent L89 A69
  constraint equal A63 A69
  constraint coincident P38 L86
  constraint coincident P38 L91
  constraint tangent L86 A70
  constraint tangent L91 A70
  constraint equal A63 A70
  constraint coincident P37 L81
  constraint coincident P37 L83
  constraint tangent L81 A71
  constraint tangent L83 A71
  constraint equal A63 A71
  constraint coincident P36 L80
  constraint coincident P36 L85
  constraint tangent L80 A72
  constraint tangent L85 A72
  constraint equal A63 A72
  constraint tangent L77 A73
  constraint tangent L79 A73
  constraint equal A63 A73
  constraint coincident P34 L75
  constraint coincident P34 L78
  constraint tangent L75 A74
  constraint tangent L78 A74
  constraint equal A63 A74
  constraint coincident P33 L74
  constraint coincident P33 L92
  constraint tangent L74 A75
  constraint tangent L92 A75
  constraint equal A63 A75
  constraint coincident P35 L76
  constraint coincident P35 L93
  constraint tangent L76 A76
  constraint tangent L93 A76
  constraint equal A63 A76
  constraint tangent L84 A77
  constraint tangent L94 A77
  constraint equal A63 A77
  constraint tangent L82 A78
  constraint tangent L95 A78
  constraint equal A63 A78
  constraint tangent L90 A79
  constraint tangent L96 A79
  constraint equal A63 A79
  constraint tangent L88 A80
  constraint tangent L97 A80
  constraint equal A63 A80
  constraint coincident P23 L41
  constraint coincident P23 L76
  constraint tangent L41 A81
  constraint tangent L76 A81
  constraint equal A63 A81
  constraint coincident L43 P25
  constraint coincident P25 L74
  constraint tangent L43 A82
  constraint equal A63 A82
  constraint coincident L40.start L84
  constraint coincident L40.start L41
  constraint tangent L84 A83
  constraint tangent L41 A83
  constraint equal A63 A83
  constraint coincident L38.start L82
  constraint coincident L38.start L39
  constraint tangent L82 A84
  constraint tangent L39 A84
  constraint equal A63 A84
  constraint coincident L37.start L90
  constraint coincident L37.start L39
  constraint tangent L90 A85
  constraint tangent L39 A85
  constraint equal A63 A85
  constraint coincident L35.start L88
  constraint coincident L35.start L48
  constraint tangent L88 A86
  constraint tangent L48 A86
  constraint equal A63 A86
  constraint coincident P0 L58
  constraint coincident P0 A0
  constraint tangent A0 A87
  constraint tangent L58 A87
  constraint coincident P2 L132
  constraint coincident P2 A2
  constraint tangent A2 A88
  constraint tangent L132 A88
  constraint tangent L9 A89
  constraint tangent L136 A89
  constraint coincident L132 P43
  constraint coincident L7 P43
  constraint tangent L132 A90
  constraint tangent L7 A90
  constraint equal A89 A90
  constraint coincident L66 P32
  constraint coincident L65 P32
  constraint tangent L66 A91
  constraint tangent L65 A91
  constraint coincident P41 L130
  constraint coincident P41 L131
  constraint tangent L130 A92
  constraint tangent L131 A92
  constraint equal A91 A92
  constraint coincident P42 L131
  constraint coincident L14 P42
  constraint tangent L131 A93
  constraint tangent L14 A93
  constraint equal A91 A93
  constraint coincident P1 L16
  constraint coincident P1 L17
  constraint tangent L16 A94
  constraint tangent L17 A94
  constraint equal A91 A94
  constraint tangent L21 A95
  constraint tangent L152 A95
  constraint tangent L156 A96
  constraint tangent L136 A96
  constraint equal A95 A96
  constraint perpendicular L46 L169
  constraint perpendicular L50 L170
  constraint perpendicular L170 L171
  constraint coincident P27 L50
  constraint coincident P27 L170
  constraint tangent L50 A98
  constraint tangent L170 A98
  constraint coincident P47 L170
  constraint coincident P47 L171
  constraint tangent L170 A99
  constraint tangent L171 A99
  constraint equal A98 A99
  constraint coincident P21 L169
  constraint tangent L46 A100
  constraint tangent L169 A100
  constraint equal A98 A100
  constraint coincident P46 L169
  constraint coincident P46 L172
  constraint tangent L169 A101
  constraint tangent L172 A101
  constraint equal A98 A101
  constraint tangent A97 A102
  constraint tangent L172 A102
  constraint equal A98 A102
  constraint tangent A97 A103
  constraint tangent L171 A103
  constraint equal A98 A103
  constraint parallel L133 L173
  constraint parallel L20 L174
  constraint parallel L19 L175
  constraint perpendicular L173 L176
  constraint parallel L0 L177
  constraint parallel L0 L178
  constraint perpendicular L177 L179
  constraint perpendicular L178 L180
  constraint coincident P40 L129
  constraint coincident L128 P40
  constraint tangent L129 A104
  constraint tangent L128 A104
  measures "d4" distance of L174.end L20.end
  measures "d16" distance of P6 P15
  measures "d19" distance of L28 L30
  measures "d21" distance of L30 L33
  measures "d22" distance of L11 L34
  measures "d24" vertical distance of P8 P12
  measures "d25" distance of P5 P11
  measures "d27" distance of P17 P20
  measures "d28" distance of P8 P12
  measures "d29" distance of P3 P9
  measures "d30" distance of L5 L6
  measures "d31" distance of S2.start P4
  measures "d33" angle of L35 L88
  measures "d34" distance of L36.end P21
  measures "d35" angle of L37 L90
  measures "d36" angle of L38 L82
  measures "d37" angle of L40 L84
  measures "d38" angle of L41 L76
  measures "d39" distance of L35.start L37.start
  measures "d40" distance of L37.start L38.start
  measures "d41" distance of L38.start L40.start
  measures "d42" distance of L40.start P23
  measures "d43" angle of L42 L74
  measures "d44" distance of P23 P25
  measures "d46" distance of P24 P25
  measures "d47" distance of L35.start P26
  measures "d49" distance of L20 L46
  measures "d50" distance of S2.end S3.start
  measures "d51" distance of S2.end P28
  measures "d52" distance of S4.end L61.start
  measures "d53" distance of P22 L61.start
  measures "d54" angle of L26 L30
  measures "d55" angle of L27 L30
  measures "d57" distance of P13 P16
  measures "d58" horizontal distance of P16 P17
  measures "d60" angle of L5 L23
  measures "d61" distance of L26 L63
  measures "d62" distance of L27 L64
  measures "d63" distance of L46 L68.start
  measures "d64" distance of L43 L68.end
  measures "d65" distance of L68.start P34
  measures "d66" distance of L69.end P35
  measures "d67" distance of L68.end P33
  measures "d68" distance of L70.start P36
  measures "d69" distance of L71.start P37
  measures "d70" distance of L72.start P38
  measures "d71" distance of L73.start P39
  measures "d72" distance of P7 P29
  measures "d73" angle of L57 L67
  measures "d74" distance of P7 P40
  measures "d75" distance of P18 P19
  measures "d76" distance of P9 P10
  measures "d77" distance of L14 L17
  measures "d80" distance of P1 L7.end
  measures "d83" distance of P3 P41
  measures "d84" distance of P2 P43
  measures "d85" distance of L33 L132
  measures "d86" distance of L21 L132
  measures "d87" distance of L58 L132
  measures "d88" distance of L58.start P44
  measures "d89" distance of L50 L133
  measures "d90" distance of P13 P14
  measures "d96" distance of P0 L9
  measures "d97" angle of L137 L138
  measures "d98" distance of L137.start L137.end
  measures "d99" distance of L138.end L139.end
  measures "d100" distance of L141.end L140.end
  measures "d101" distance of L139.end L140.end
  measures "d102" distance of L141.end L142.end
  measures "d103" angle of L139 L140
  measures "d104" distance of L143.end L142.end
  measures "d105" angle of L145 L146
  measures "d106" angle of L148 L149
  measures "d107" distance of L137.start L148.end
  measures "d108" angle of L150 L151
  measures "d109" distance of L148.end L150.end
  measures "d110" distance of L66 L146.end
  measures "d111" distance of P31 P32
  measures "d112" distance of L23 L65
  measures "d113" distance of P41 P42
  measures "d114" distance of L0 L65
  measures "d115" angle of L48 L49
  measures "d116" distance of L147 L154
  measures "d118" distance of L145.end L144.end
  measures "d119" distance of L144.end L143.end
  measures "d120" distance of L145.end L146.end
  measures "d121" angle of L141 L142
  measures "d122" angle of L138 L139
  measures "d123" distance of L137.end L138.end
  measures "d124" angle of L137 L148
  measures "d125" angle of L146 L147
  measures "d127" radius of A4
  measures "d129" radius of A26
  measures "d130" radius of A27
  measures "d131" radius of A32
  measures "d132" radius of A33
  measures "d133" radius of A34
  measures "d134" radius of A35
  measures "d135" radius of A60
  measures "d136" radius of A61
  measures "d137" radius of A62
  measures "d138" radius of A63
  measures "d139" radius of A87
  measures "d140" radius of A88
  measures "d141" radius of A89
  measures "d142" radius of A91
  measures "d143" radius of A95
  measures "d145" distance of P21 P46
  measures "d146" distance of P27 P47
  measures "d148" diameter of A97
  measures "d150" radius of A98
  measures "d164" radius of A9
  measures "d165" radius of A104
  measures "d166" radius of A7
  measures "d167" radius of A8
  measures "d168" radius of A6
extrude "Extrude1" add sketch "Sketch1" along normal blind 5